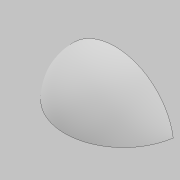
# Autodesk Inventor part: cover2_cap_extended
Saved by Autodesk Inventor 2021 (Build 250183000, 183)
## iProperties
Created: 2021-06-01
Part Number: cover2_cap_extended
Material: Generic
Document SubType Name: Modeling
Designer: Watchdog
Density: 1 g/cm^3
Appearance: Default
Author: Watchdog
Autodesk Inventor part; units mm, degrees
ref_plane "XZ Plane" through (0, 0, 0) normal (0, 1, 0) x (-1, 0, 0)
ref_plane "XY Plane" through (0, 0, 0) normal (0, 0, 1) x (1, 0, 0)
sketch "Sketch1" plane through (0, 0, 0) normal (0, 0, 1) x (1, 0, 0)
  arc A0 (0, 900) -> (-1039.2305, 0) centre (0, -150) ccw
  arc A1 (1039.2305, 0) -> (0, 900) centre (0, -150) ccw
  arc A2 (0, 890) -> (-1029.1258, 0) centre (0, -150) ccw
  arc A3 (1029.1258, 0) -> (0, 890) centre (0, -150) ccw
  line L0 (1029.1258, 0) -> (1039.2305, 0)
  line L1 (-1039.2305, 0) -> (-1029.1258, 0)
  point P0 (0, 0)
  dimension "d0" = 0
  dimension "d1" = 0
  dimension "d2" = 0
  dimension "d3" = 150
  dimension "d6" = 900
  dimension "d8" = 1039.2305
  dimension "d10" = 0
  dimension "d11" = 10
  dimension "d12" = 0
  constraints: 8 point on circle, 4 centre point, 4 end point, 2 horizontal, 1 coincident, 1 other
  measures "d0" vertical distance of point (0, 0) L1.start
  measures "d1" horizontal distance of point (0, 0) A0.start
  measures "d2" horizontal distance of point (0, 0) A0.centre
  measures "d3" distance of point (0, 0) A0.centre
  measures "d6" distance of point (0, 0) A0.start
  measures "d8" distance of point (0, 0) L1.start
  measures "d10" vertical distance of point (0, 0) L0.end
  measures "d11" radial gap between concentric circles of A0 A2
  measures "d12" horizontal distance of A0.start A2.start
revolve "Revolution2" add sketch "Sketch1" angle 90 about axis through (1029.1258, 0, 0) along (1, 0, 0)
ref_plane "end1" through (1039.2305, 0, 0) normal (1, 0, 0) x (0, 1, 0)
ref_plane "end2" through (-1039.2305, 0, 0) normal (1, 0, 0) x (0, 1, 0)
body "Solid2"
